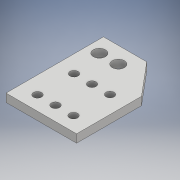
# Autodesk Inventor part: Wheels
Saved by Autodesk Inventor 2017 (Build 210142000, 142)
## iProperties
Created: 2016-12-07
Part Number: Wheels
Material: Generic
Document SubType Name: Modeling
Designer: umr
Density: 1 g/cm^3
Appearance: Default
Author: umr
Autodesk Inventor part; units mm, degrees
ref_plane "YZ Plane" through (0, 0, 0) normal (1, 0, 0) x (0, 1, 0)
ref_plane "XZ Plane" through (0, 0, 0) normal (0, 1, 0) x (-1, 0, 0)
ref_plane "XY Plane" through (0, 0, 0) normal (0, 0, 1) x (1, 0, 0)
sketch "Sketch1" plane through (0, 0, 0) normal (0, 0, 1) x (1, 0, 0)
  line L0 (0, 0) -> (86.8973, 0)
  line L1 (53.3333, 120) -> (0, 120)
  line L2 (0, 120) -> (0, 0)
  line L3 (86.8973, 0) -> (86.8973, 80)
  line L4 (53.3333, 120) -> (86.8973, 80)
  dimension "d0" = 120
  dimension "d2" = 53.3333
  dimension "d6" = 90
  dimension "d9" = 130
  dimension "d10" = 90
  dimension "d11" = 80
  constraints: 10 end point, 1 horizontal, 1 parallel
  measures "d0" distance of L1.end L0.start
  measures "d2" distance of L1.start L1.end
  measures "d6" angle of L0 L2
  measures "d9" angle of L4 L1
  measures "d10" angle of L0 L3
  measures "d11" distance of L0.end L3.end
extrude "Extrusion1" add sketch "Sketch1" along normal blind 10
sketch "Sketch2" plane through (0, 0, 10) normal (0, 0, 1) x (1, 0, 0)
  line L0 (86.8973, 0) -> (86.8973, 80) projected
  line L1 (86.8973, 40) -> (0, 40)
  line L2 (0, 120) -> (0, 0) projected
  circle A0 centre (21.2374, 62.5) radius 5
  circle A1 centre (43.4487, 62.5) radius 5
  circle A2 centre (65.6599, 62.5) radius 5
  circle A3 centre (21.2374, 17.5) radius 5
  circle A4 centre (43.4487, 17.5) radius 5
  circle A5 centre (65.6599, 17.5) radius 5
  line L3 (0, 0) -> (86.8973, 0) projected
  circle A6 centre (15, 100) radius 7.5
  line L4 (53.3333, 120) -> (0, 120) projected
  circle A7 centre (38.3333, 100) radius 7.5
  dimension "d12" = 10
  dimension "d13" = 80
  dimension "d16" = 21.2374
  dimension "d17" = 22.5
  dimension "d20" = 22.2113
  dimension "d23" = 45
  dimension "d28" = 45
  dimension "d30" = 86.8973
  dimension "d31" = 20
  dimension "d32" = 15
  dimension "d33" = 15
  dimension "d34" = 20
  dimension "d35" = 15
  dimension "d36" = 53.3333
  dimension "d37" = 15
  constraints: 8 centre point, 2 end point, 2 horizontal, 1 midpoint, 1 point on line, 1 vertical, 10 other
  measures "d12" diameter of A0
  measures "d13" distance of L0.start L0.end
  measures "d16" distance from line of L2 A0.centre
  measures "d17" distance from line of L1 A0.centre
  measures "d20" distance of A0.centre A1.centre
  measures "d23" distance of A0.centre A3.centre
  measures "d28" distance of A5.centre A2.centre
  measures "d30" distance of L1.start L1.end
  measures "d31" distance from line of L4 A6.centre
  measures "d32" diameter of A6
  measures "d33" diameter of A7
  measures "d34" distance from line of A7.centre L4
  measures "d35" distance from line of L2 A6.centre
  measures "d36" distance of L4.start L2.start
  measures "d37" horizontal distance of L4.start A7.centre
extrude "Extrusion2" cut sketch "Sketch2" against normal up to next contours A0 | A1 | A2 | A3 | A4 | A5 | A6 | A7
equation "\"d2\" = 0.666667 * d11"
equation "\"d11\" = 0.666667 * d0"
equation "\"d16\" = 0.1 * d15"
equation "\"d20\" = -d16 + 0.5 * d30"
equation "\"d23\" = 2 * d17"
equation "\"d33\" = d32"
equation "\"d34\" = d31"
equation "\"d15\" = 212.373871"
body "Solid1"
